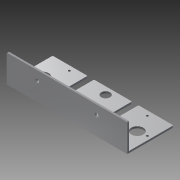
# Autodesk Inventor part: drzak_motory
Saved by Autodesk Inventor 2015 (Build 190159000, 159)
## iProperties
Created: 2012-08-21
Part Number: drzak_motory
Material: Generic
Document SubType Name: Modeling
Designer: idle-rug
Density: 1 g/cm^3
Appearance: Default
Author: idle-rug
Autodesk Inventor part; units mm, degrees
ref_plane "YZ Plane" through (0, 0, 0) normal (1, 0, 0) x (0, 1, 0)
ref_plane "XZ Plane" through (0, 0, 0) normal (0, 1, 0) x (-1, 0, 0)
ref_plane "XY Plane" through (0, 0, 0) normal (0, 0, 1) x (1, 0, 0)
sketch "Sketch1" plane through (0, 0, 0) normal (1, 0, 0) x (0, 1, 0)
  line L0 (-25, 24) -> (-25, -24)
  line L1 (-25, -24) -> (25, -24)
  line L2 (25, -24) -> (25, -22)
  line L3 (25, -22) -> (-23, -22)
  line L4 (-23, -22) -> (-23, 24)
  line L5 (-23, 24) -> (-25, 24)
  constraints: 12 end point, 2 perpendicular, 1 parallel
extrude "Extrusion1" add sketch "Sketch1" along normal mid plane 131
sketch "Sketch2" plane through (65.5, 25, -24) normal (0, 0, -1) x (-1, 0, 0)
  circle A0 centre (41.4, -25) radius 3.5
  circle A1 centre (89.6, -25) radius 3.5
  line L0 (131, 0) -> (0, 0) projected
  line L1 (37.9, -25) -> (44.9, -25)
  line L2 (44.9, -25) -> (44.9, 0)
  line L3 (44.9, 0) -> (37.9, 0)
  line L4 (37.9, 0) -> (37.9, -25)
  line L5 (86.1, -25) -> (93.1, -25)
  line L6 (93.1, -25) -> (93.1, 0)
  line L7 (93.1, 0) -> (86.1, 0)
  line L8 (86.1, 0) -> (86.1, -25)
  line L9 (65.5, 0) -> (65.5, -8)
  circle A2 centre (65.5, -8) radius 4.75
  dimension "d17" = 7
  dimension "d18" = 7
  dimension "d129" = 8
  dimension "d130" = 9.5
  constraints: 18 end point, 4 parallel, 3 point on line, 2 horizontal, 2 horizontal alignment, 2 perpendicular, 1 centre point, 1 coincident, 1 midpoint, 1 vertical, 4 other
  measures "d129" distance of L9.start L9.end
  measures "d130" diameter of A2
hole "Hole1" at (24.1, 0, -24) at (-24.1, 0, -24) direction (0, 0, 1) diameter 7 depth 2
sketch "Sketch3" plane through (65.5, 25, -24) normal (0, 0, -1) x (-1, 0, 0)
  line L0 (65.5, -25) -> (14.2, -25)
  line L1 (65.5, -25) -> (116.8, -25)
  circle A0 centre (14.2, -25) radius 9.5
  circle A1 centre (14.2, -25) radius 1.75
  circle A2 centre (116.8, -25) radius 1.75
  dimension "d26" = 51.3
  dimension "d27" = 51.3
  dimension "d28" = 19
  dimension "d29" = 3.5
  dimension "d30" = 3.5
  constraints: 4 end point, 3 centre point, 3 coincident, 1 collinear, 1 horizontal
  measures "d26" distance of L0.start L0.end
  measures "d27" distance of L0.start L1.end
  measures "d28" diameter of A0
  measures "d29" diameter of A1
  measures "d30" diameter of A2
hole "Hole2" at (51.3, 0, -24) at (-51.3, 0, -24) direction (0, 0, 1) diameter 3.5 depth 2
sketch "Sketch7" plane through (65.5, 25, -24) normal (0, 0, -1) x (-1, 0, 0)
  circle A0 centre (14.2, -25) radius 1.75 projected
  circle A1 centre (14.2, -25) radius 3.5
  point P0 (65.5, -25)
  dimension "d89" = 7
  constraints: 1 centre point, 1 coincident
  measures "d89" diameter of A1
extrude "Extrusion3" cut sketch "Sketch7" against normal blind 2
sketch "Sketch8" plane through (65.5, 25, -24) normal (0, 0, -1) x (-1, 0, 0)
  circle A0 centre (14.2, -25) radius 3.5 projected
  line L0 (14.2, -25) -> (39.2, -25) construction
  circle A1 centre (19.1497, -20.0503) radius 18.4
  circle A2 centre (19.1497, -20.0503) radius 15.5
  line L1 (14.2, -25) -> (19.1497, -20.0503)
  line L2 (19.1497, -20.0503) -> (36.8274, -2.3726)
  line L3 (36.8274, -2.3726) -> (1.4721, -37.7279)
  line L4 (6.139, -7.0395) -> (32.1605, -33.061)
  circle A3 centre (8.1896, -9.0901) radius 1.2
  circle A4 centre (30.1099, -31.0104) radius 1.2
  circle A5 centre (23.1614, -5.0784) radius 1.2
  circle A6 centre (4.1779, -24.0619) radius 1.2
  circle A7 centre (15.1381, -35.0221) radius 1.2
  circle A8 centre (34.1216, -16.0386) radius 1.2
  point P0 (65.5, -25)
  dimension "d96" = 31
  dimension "d97" = 25
  dimension "d98" = 180
  dimension "d99" = 50
  dimension "d100" = 2.4
  dimension "d101" = 2.4
  dimension "d104" = 2.4
  dimension "d105" = 2.4
  dimension "d106" = 2.4
  dimension "d107" = 2.4
  constraints: 10 end point, 8 centre point, 8 point on circle, 2 coincident, 2 collinear, 2 point on line, 1 horizontal, 1 perpendicular
  measures "d96" diameter of A2
  measures "d97" distance of L1.end L2.end
  measures "d98" angle of L2 L1
  measures "d99" distance of L2.end L3.end
  measures "d100" diameter of A3
  measures "d101" diameter of A4
  measures "d104" diameter of A5
  measures "d105" diameter of A6
  measures "d106" diameter of A7
  measures "d107" diameter of A8
extrude "Extrusion4" cut sketch "Sketch8" against normal blind 2 contours A3 A2 L4 | L4 A2 A3 | A4 A2 L4 | L4 A2 A4 | A6 A2 | A2 A6 | A7 A2 | A2 A7 | A8 A2 | A2 A8 | A5 A2 | A2 A5 | L4 A3 A2 | A2 A3 L4 | L4 A4 A2 | A2 A4 L4
sketch "Sketch9" plane through (65.5, 25, -24) normal (0, 0, -1) x (-1, 0, 0)
  circle A0 centre (34.1216, -16.0386) radius 1.2 projected
  circle A1 centre (8.1896, -9.0901) radius 1.2 projected
  circle A2 centre (15.1381, -35.0221) radius 1.2 projected
  point P0 (65.5, -25)
extrude "Extrusion6" add sketch "Sketch9" against normal blind 2
sketch "Sketch11" plane through (65.5, 25, -24) normal (0, 0, -1) x (-1, 0, 0)
  circle A0 centre (4.1779, -24.0619) radius 1.2 projected
  circle A1 centre (30.1099, -31.0104) radius 1.2 projected
  circle A2 centre (23.1614, -5.0784) radius 1.2 projected
  circle A3 centre (14.2, -25) radius 3.5 projected
  circle A4 centre (116.8, -25) radius 1.75 projected
  line L0 (65.5, -25) -> (65.5, 0)
  line L1 (0, 0) -> (131, 0) projected
  circle A5 centre (126.8221, -24.0619) radius 1.2
  circle A6 centre (100.8901, -31.0104) radius 1.2
  circle A7 centre (107.8386, -5.0784) radius 1.2
  circle A8 centre (116.8, -25) radius 3.5
  constraints: 4 centre point, 4 symmetric about line, 2 end point, 1 midpoint, 4 other
extrude "Extrusion7" cut sketch "Sketch11" against normal blind 2 contours A5 | A6 | A7 | A8
sketch "Sketch12" plane through (65.5, 25, -24) normal (0, 0, -1) x (-1, 0, 0)
  circle A0 centre (116.8, -25) radius 3.5 projected
  circle A1 centre (14.2, -25) radius 3.5 projected
  circle A2 centre (14.2, -25) radius 6.5
  circle A3 centre (116.8, -25) radius 6.5
  point P0 (65.5, -25)
  dimension "d116" = 13
  dimension "d117" = 13
  constraints: 2 centre point, 2 coincident
  measures "d116" diameter of A2
  measures "d117" diameter of A3
extrude "Extrusion8" cut sketch "Sketch12" against normal blind 2
extrude "Extrusion9" cut sketch "Sketch2" against normal blind 2 contours L1 A0 | L0 L6 A1 L8 | A0 L1 | A0 L4 L0 L2 | L5 A1 | A1 L5
fillet "Fillet1" radius 1 4 edges at (20.6, 25, -23) (27.6, 25, -23) (-20.6, 25, -23) (-27.6, 25, -23)
fillet "Fillet2" radius 1 2 edges at (65.5, 25, -23) (-65.5, 25, -23)
extrude "Extrusion10" cut sketch "Sketch2" against normal blind 2 contours A2
sketch "Sketch14" plane through (-65.5, -25, 24) normal (0, 0, 1) x (1, 0, 0)
  line L0 (0, 2) -> (131, 2)
  line L1 (131, 2) -> (131, 0)
  line L2 (131, 0) -> (0, 0)
  line L3 (0, 0) -> (0, 2)
  point P0 (65.5, 25)
  constraints: 8 end point, 2 parallel, 1 horizontal, 1 perpendicular
extrude "Extrusion11" cut sketch "Sketch14" against normal blind 18
fillet "Fillet3" radius 1 2 edges at (-65.5, -24, 6) (65.5, -24, 6)
sketch "Sketch15" plane through (-65.5, -25, -24) normal (0, -1, 0) x (1, 0, 0)
  circle A0 centre (97.65, 20) radius 2
  circle A1 centre (33.35, 20) radius 2
  point P0 (65.5, 24)
  point P1 (131, 0)
  point P2 (0, 0)
  dimension "d139" = 4
  dimension "d140" = 4
  constraints: 2 centre point
  measures "d139" diameter of A0
  measures "d140" diameter of A1
extrude "Extrusion12" cut sketch "Sketch15" against normal blind 2
body "Solid1"
